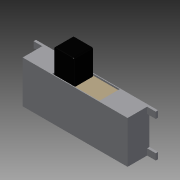
# Autodesk Inventor part: msk12c02
Saved by Autodesk Inventor 2014 SP1 (Build 180222100, 222)
## iProperties
Created: 2023-06-06
Part Number: msk12c02
Material: Типовые
Document SubType Name: Modeling
Designer: Alex
Density: 1 g/cm^3
Appearance: По умолчанию
Author: Alex
Autodesk Inventor part; units mm, degrees
ref_plane "YZ Plane" through (0, 0, 0) normal (1, 0, 0) x (0, 1, 0)
ref_plane "XZ Plane" through (0, 0, 0) normal (0, 1, 0) x (-1, 0, 0)
ref_plane "XY Plane" through (0, 0, 0) normal (0, 0, 1) x (1, 0, 0)
sketch "Эскиз1" plane through (0, 0, 0) normal (0, 1, 0) x (-1, 0, 0)
  line L0 (0, 0) -> (6.7, 0)
  line L1 (6.7, 0) -> (6.7, 2.7)
  line L2 (6.7, 2.7) -> (0, 2.7)
  line L3 (0, 2.7) -> (0, 0)
  dimension "d0" = 6.7
  dimension "d1" = 2.7
  constraints: 8 end point, 2 parallel, 1 horizontal, 1 perpendicular
  measures "d0" distance of L2.end L1.end
  measures "d1" distance of L1.end L0.end
extrude "Выдавливание1" add sketch "Эскиз1" against normal blind 1.4
sketch "Эскиз2" plane through (0, 0, 0) normal (0, 1, 0) x (1, 0, 0)
  line L0 (0, 0) -> (-6.7, 0) projected
  circle A0 centre (-4.85, -1.35) radius 0.35
  circle A1 centre (-1.85, -1.35) radius 0.35
  point P0 (0, -2.7)
  dimension "d4" = 0.7
  dimension "d6" = 1.35
  dimension "d7" = 2.7
  dimension "d9" = 1.35
  dimension "d10" = 3
  dimension "d11" = 1.85
  dimension "d12" = 6.7
  constraints: 2 centre point, 1 equal radius
  measures "d4" diameter of A0
  measures "d6" distance from line of L0 A0.centre
  measures "d7" distance of point (0, -2.7) L0.start
  measures "d9" distance from line of L0 A1.centre
  measures "d10" distance of A1.centre A0.centre
  measures "d11" horizontal distance of L0.end A0.centre
  measures "d12" distance of L0.start L0.end
extrude "Выдавливание2" add sketch "Эскиз2" along normal blind 0.5
sketch "Эскиз3" plane through (-6.7, 0, 2.7) normal (0, 0, 1) x (1, 0, 0)
  line L0 (0, 0) -> (6.7, 0) projected
  line L1 (1.9, -0.05) -> (3.2, -0.05)
  line L2 (3.2, -0.05) -> (3.2, -1.35)
  line L3 (3.2, -1.35) -> (1.9, -1.35)
  line L4 (1.9, -1.35) -> (1.9, -0.05)
  line L5 (1.85, -0.05) -> (4.85, -0.05)
  line L6 (4.85, -0.05) -> (4.85, -1.35)
  line L7 (4.85, -1.35) -> (1.85, -1.35)
  line L8 (1.85, -1.35) -> (1.85, -0.05)
  line L9 (3.5, -0.05) -> (4.8, -0.05)
  line L10 (4.8, -0.05) -> (4.8, -1.35)
  line L11 (4.8, -1.35) -> (3.5, -1.35)
  line L12 (3.5, -1.35) -> (3.5, -0.05)
  point P0 (0, -1.4)
  point P1 (6.7, -1.4)
  dimension "d15" = 1.3
  dimension "d16" = 1.3
  dimension "d18" = 0.05
  dimension "d20" = 3
  dimension "d21" = 1.3
  dimension "d22" = 1.85
  dimension "d23" = 6.7
  dimension "d24" = 0.05
  dimension "d25" = 0.05
  dimension "d51" = 1.3
  dimension "d52" = 1.3
  dimension "d53" = 0.05
  constraints: 24 end point, 6 parallel, 3 horizontal, 3 perpendicular
  measures "d15" distance of L2.end L3.end
  measures "d16" distance of L1.end L2.end
  measures "d18" distance between parallel lines of L0 L1
  measures "d20" distance of L6.end L7.end
  measures "d21" distance of L5.end L6.end
  measures "d22" distance from line of L8 L0.start
  measures "d23" distance of point (6.7, -1.4) point (0, -1.4)
  measures "d24" distance between parallel lines of L0 L5
  measures "d25" distance between parallel lines of L8 L4
  measures "d51" distance of L10.end L11.end
  measures "d52" distance of L9.end L10.end
  measures "d53" distance between parallel lines of L10 L6
extrude "Выдавливание3" add sketch "Эскиз3" along normal blind 1.5 contours L1 L2 L3 L4
sketch "Эскиз4" plane through (0, 0, 0) normal (0, 1, 0) x (1, 0, 0)
  line L0 (0, 0) -> (0.55, 0)
  line L1 (0.55, 0) -> (0.55, -0.4)
  line L2 (0.55, -0.4) -> (0, -0.4)
  line L3 (0, -0.4) -> (0, 0)
  line L4 (0, -2.7) -> (0.55, -2.7)
  line L5 (0.55, -2.7) -> (0.55, -2.3)
  line L6 (0.55, -2.3) -> (0, -2.3)
  line L7 (0, -2.3) -> (0, -2.7)
  line L8 (-6.7, -2.7) -> (-7.25, -2.7)
  line L9 (-7.25, -2.7) -> (-7.25, -2.3)
  line L10 (-7.25, -2.3) -> (-6.7, -2.3)
  line L11 (-6.7, -2.3) -> (-6.7, -2.7)
  line L12 (-6.7, 0) -> (-7.25, 0)
  line L13 (-7.25, 0) -> (-7.25, -0.4)
  line L14 (-7.25, -0.4) -> (-6.7, -0.4)
  line L15 (-6.7, -0.4) -> (-6.7, 0)
  dimension "d28" = 0.55
  dimension "d29" = 0.4
  dimension "d30" = 0.4
  dimension "d31" = 0.55
  dimension "d32" = 0.4
  dimension "d33" = 0.4
  constraints: 32 end point, 8 parallel, 4 horizontal, 4 perpendicular
  measures "d28" distance of L1.end L2.end
  measures "d29" distance of L0.end L1.end
  measures "d30" distance of L5.end L4.end
  measures "d31" distance of L9.end L10.end
  measures "d32" distance of L8.end L9.end
  measures "d33" distance of L13.end L12.end
extrude "Выдавливание4" add sketch "Эскиз4" against normal blind 0.15
fillet "Сопряжение1" radius 0.1 2 edges at (-5.2, 0.5, 1.35) (-2.2, 0.5, 1.35)
fillet "Сопряжение2" radius 0.1 8 edges at (-4.8, -0.05, 3.45) (-3.5, -0.05, 3.45) (-4.15, -0.05, 4.2) (-4.15, -1.35, 4.2) (-3.5, -0.7, 4.2) (-3.5, -1.35, 3.45) (-4.8, -1.35, 3.45) (-4.8, -0.7, 4.2)
fillet "Сопряжение2" radius 0.1 2 edges at (-4.15, -0.05, 4.2) (-4.15, -1.35, 4.2)
sketch "Эскиз6" plane through (-6.7, -1.4, 2.7) normal (0, 0, 1) x (1, 0, 0)
  line L0 (3.2, 1.25) -> (3.2, 0.15) projected
  arc A0 (3.1, 0.05) -> (3.2, 0.15) centre (3.1, 0.15) ccw projected
  arc A1 (1.9, 0.15) -> (2, 0.05) centre (2, 0.15) ccw projected
  line L1 (1.9, 0.15) -> (1.9, 1.25) projected
  arc A2 (2, 1.35) -> (1.9, 1.25) centre (2, 1.25) ccw projected
  arc A3 (3.2, 1.25) -> (3.1, 1.35) centre (3.1, 1.25) ccw projected
  line L2 (0, 0) -> (6.7, 0)
  line L3 (1.85, 1.35) -> (4.85, 1.35) projected
  line L4 (4.85, 1.35) -> (4.85, 0.05) projected
  line L5 (1.85, 0.05) -> (1.85, 1.35) projected
  line L6 (4.85, 0.05) -> (1.85, 0.05) projected
  constraints: 2 end point
extrude "Выдавливание5" cut sketch "Эскиз6" against normal blind 0.1 contours A3 L3 L4 L6 A0 L0 | A2 L1 A1 L6 L5 L3
sketch "Эскиз7" plane through (0, 0, 0) normal (0, 1, 0) x (1, 0, 0)
  circle A0 centre (-4.85, -1.35) radius 0.35 projected
  circle A1 centre (-1.85, -1.35) radius 0.35 projected
  line L0 (0.55, 0) -> (-7.25, 0) projected
  line L1 (-7.25, 0) -> (-7.25, -0.4) projected
  line L2 (-7.25, -0.4) -> (-6.7, -0.4) projected
  line L3 (-6.7, -0.4) -> (-6.7, -2.3) projected
  line L4 (-6.7, -2.3) -> (-7.25, -2.3) projected
  line L5 (-7.25, -2.3) -> (-7.25, -2.7) projected
  line L6 (-7.25, -2.7) -> (0.55, -2.7) projected
  line L7 (0.55, -2.7) -> (0.55, -2.3) projected
  line L8 (0.55, -2.3) -> (0, -2.3) projected
  line L9 (0, -2.3) -> (0, -0.4) projected
  line L10 (0, -0.4) -> (0.55, -0.4) projected
  line L11 (0.55, -0.4) -> (0.55, 0) projected
  point P0 (0, 0)
  dimension "d49" = 1.35
  dimension "d50" = 3
  measures "d49" distance from line of L6 A0.centre
  measures "d50" distance of A1.centre A0.centre
sketch "Эскиз8" plane through (-6.7, -1.4, 2.7) normal (0, 0, 1) x (1, 0, 0)
  line L0 (1.85, 1.35) -> (2, 1.35) projected
  line L1 (2, 1.35) -> (3.1, 1.35) projected
  line L2 (3.1, 1.35) -> (2, 1.35) projected
  line L3 (3.6, 1.35) -> (4.7, 1.35) projected
  line L4 (1.85, 1.35) -> (4.85, 1.35) projected
  line L5 (4.85, 1.35) -> (4.85, 0.05) projected
  line L6 (4.85, 0.05) -> (3.1, 0.05) projected
  line L7 (4.7, 0.05) -> (3.6, 0.05) projected
  line L8 (4.85, 0.05) -> (3.1, 0.05) projected
  line L9 (3.1, 0.05) -> (2, 0.05) projected
  line L10 (2, 0.05) -> (1.85, 0.05) projected
  line L11 (1.85, 0.05) -> (1.85, 1.35) projected
equation "\"d6\" = 0.5 * d7"
equation "\"d9\" = d6"
equation "\"d11\" = -0.5 * d10 + 0.5 * d12"
equation "\"d22\" = -0.5 * d20 + 0.5 * d23"
